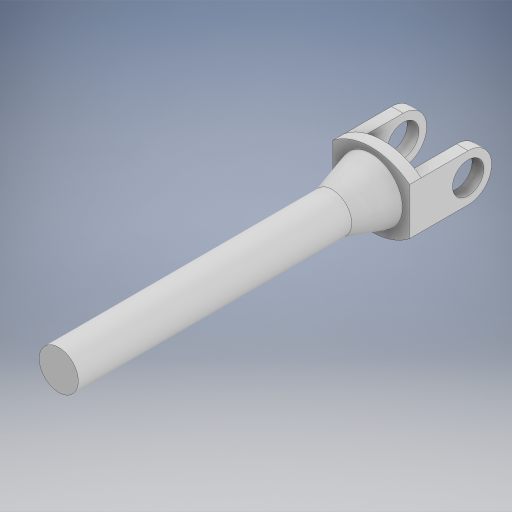
# Autodesk Inventor part: wheel hub
Saved by Autodesk Inventor 2024 (Build 280153000, 153)
## iProperties
Created: 2024-04-03
Part Number: wheel hub
Material: Generic
Document SubType Name: Modeling
Designer: Alex
Density: 1 g/cm^3
Appearance: Default
Author: Alex
Autodesk Inventor part; units mm, degrees
ref_plane "YZ Plane" through (0, 0, 0) normal (1, 0, 0) x (0, 1, 0)
ref_plane "XZ Plane" through (0, 0, 0) normal (0, 1, 0) x (-1, 0, 0)
sketch "Sketch1" plane through (0, 0, 0) normal (0, 0, 1) x (1, 0, 0)
  circle A0 centre (0, 0) radius 11.5
  constraints: 1 centre point, 1 coincident
extrude "Extrusion1" add sketch "Sketch1" against normal blind 3
sketch "Sketch2" plane through (0, 0, -3) normal (0, 0, -1) x (-1, 0, 0)
  line L0 (-9.8107, 6) -> (-6.8107, 6)
  line L1 (-6.8107, 6) -> (-6.8107, -6)
  line L2 (-6.8107, -6) -> (-9.8107, -6)
  line L3 (-9.8107, -6) -> (-9.8107, 6)
  line L4 (6.8107, 6) -> (9.8107, 6)
  line L5 (9.8107, 6) -> (9.8107, -6)
  line L6 (9.8107, -6) -> (6.8107, -6)
  line L7 (6.8107, -6) -> (6.8107, 6)
  circle A0 centre (0, 0) radius 11.5 construction
  line L8 (0, 11.5) -> (0, -11.5) construction
  arc A1 (-9.8107, 6) -> (-9.8107, -6) centre (0, 0) ccw
  arc A2 (9.8107, -6) -> (9.8107, 6) centre (0, 0) ccw
  arc A3 (9.8107, 6) -> (-9.8107, 6) centre (0, -6.6392) ccw
  arc A4 (-9.8107, -6) -> (9.8107, -6) centre (0, 6.6392) ccw
  circle A5 centre (0, 0) radius 11.5
  point P0 (6.8107, 0)
  dimension "d18" = 3
  dimension "d19" = 12
  dimension "d29" = 16
  constraints: 18 end point, 11 point on circle, 5 centre point, 4 parallel, 2 coincident, 2 concentric, 2 equal length, 2 equal radius, 2 horizontal, 2 horizontal alignment, 2 midpoint, 2 perpendicular, 1 point on line, 1 vertical, 1 other
  measures "d18" distance of L4.start L4.end
  measures "d19" distance of L4.end L5.end
  measures "d29" radius of A4
extrude "Extrusion4" add sketch "Sketch2" along normal blind 18 contours L0 L1 L2 L3 | L5 L6 L7 L4
fillet "Fillet3" radius 6 4 edges at (8.3107, 6, -21) (8.3107, -6, -21) (-8.3107, 6, -21) (-8.3107, -6, -21)
sketch "Sketch3" plane through (9.8107, -6, -3) normal (1, 0, 0) x (0, 0, -1)
  arc A0 (12, 0) -> (12, 12) centre (12, 6) ccw construction
  circle A1 centre (12, 6) radius 4
  point P0 (-3, 6)
  dimension "d23" = 8
  constraints: 1 centre point, 1 coincident
  measures "d23" diameter of A1
extrude "Extrusion5" cut sketch "Sketch3" against normal through all
extrude "Extrusion6" cut sketch "Sketch2" against normal blind 10 contours L3 A1 | A5 A3 | A4 A5 | A2 L5
sketch "Sketch5" plane through (0, 0, 0) normal (0, 0, 1) x (1, 0, 0)
  circle A0 centre (0, 0) radius 8
  dimension "d35" = 16
  constraints: 1 centre point, 1 coincident
  measures "d35" diameter of A0
ref_plane "Work Plane1" through (0, 0, 10) normal (0, 0, 1) x (1, 0, 0)
sketch "Sketch6" plane through (0, 0, 10) normal (0, 0, 1) x (1, 0, 0)
  circle A0 centre (0, 0) radius 8 construction
  circle A1 centre (0, 0) radius 5
  dimension "d37" = 10
  constraints: 1 centre point, 1 coincident
  measures "d37" diameter of A1
loft "Loft1" add profiles "Sketch5", "Sketch6"
sketch "Sketch7" plane through (0, 0, 10) normal (0, 0, 1) x (1, 0, 0)
  circle A0 centre (0, 0) radius 5
  circle A1 centre (0, 0) radius 5 construction
  constraints: 1 centre point, 1 coincident, 1 concentric
extrude "Extrusion8" add sketch "Sketch7" along normal blind 70
body "Solid1"
